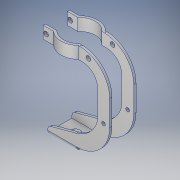
# Autodesk Inventor part: ARM
Saved by Autodesk Inventor 2018 (Build 220112000, 112)
## iProperties
Created: 2018-02-23
Part Number: ARM
Material: Aluminum 6061
Document SubType Name: Modeling
Designer: 238438
Density: 2.7 g/cm^3
Appearance: Aluminum - Flat
Mass: 2.14686 g
Surface Area: 19.7952 cm^2
Volume: 0.795133 cm^3
Author: 238438
Autodesk Inventor part; units mm, degrees
ref_plane "YZ Plane" through (0, 0, 0) normal (1, 0, 0) x (0, 1, 0)
ref_plane "XZ Plane" through (0, 0, 0) normal (0, 1, 0) x (-1, 0, 0)
ref_plane "XY Plane" through (0, 0, 0) normal (0, 0, 1) x (1, 0, 0)
sketch "Sketch1" plane through (0, 0, 0) normal (0, 1, 0) x (-1, 0, 0)
  line L0 (0, 0) -> (-12.0269, 0)
  line L1 (-12.0269, 0) -> (-12.0269, -11.1252)
  line L2 (-12.0269, -11.1252) -> (0, -11.1252)
  line L3 (0, -11.1252) -> (0, 0)
  circle A0 centre (-6.0198, -5.5626) radius 1.9876
  dimension "d0" = 12.0269
  dimension "d1" = 11.1252
  dimension "d2" = 5.5626
  dimension "d3" = 6.0198
  dimension "d4" = 3.9751
  constraints: 8 end point, 2 parallel, 1 centre point, 1 coincident, 1 horizontal, 1 perpendicular
  measures "d0" distance of L2.end L1.end
  measures "d1" distance of L1.end L0.end
  measures "d2" distance from line of L0 point (-6.02, -5.563)
  measures "d3" distance from line of L3 point (-6.02, -5.563)
  measures "d4" diameter of A0
extrude "Extrusion1" add sketch "Sketch1" along normal blind 0.9652
sketch "Sketch2" plane through (0, 0.9652, 0) normal (0, 1, 0) x (1, 0, 0)
  line L0 (0, 11.1252) -> (0, 0) projected
  line L1 (12.0269, 0) -> (12.0269, 11.1252) projected
  line L2 (0, 0) -> (12.0269, 0)
  line L3 (12.0269, 0) -> (12.0269, 0.9779)
  line L4 (12.0269, 0.9779) -> (0, 0.9779)
  line L5 (0, 0.9779) -> (0, 0)
  line L6 (12.0269, 11.1252) -> (0, 11.1252) projected
  line L7 (12.0269, 11.1252) -> (0, 11.1252)
  line L8 (0, 11.1252) -> (0, 10.1473)
  line L9 (0, 10.1473) -> (12.0269, 10.1473)
  line L10 (12.0269, 10.1473) -> (12.0269, 11.1252)
  dimension "d7" = 0.9779
  dimension "d8" = 0.9779
  constraints: 16 end point, 4 parallel, 2 horizontal, 2 perpendicular, 2 point on line
  measures "d7" distance of L3.end L2.end
  measures "d8" distance of L8.end L7.end
extrude "Extrusion2" add sketch "Sketch2" along normal blind 12.7 contours L6 L1 L9 L0 | L4 L1 L2 L0
sketch "Sketch3" plane through (0, 0, 0) normal (0, 0, 1) x (1, 0, 0)
  line L0 (0, 0.9652) -> (0, 13.6652) projected
  line L1 (0, 3.302) -> (12.0269, 6.5246)
  line L2 (12.0269, 0.9652) -> (12.0269, 13.6652) projected
  line L3 (0, 3.302) -> (12.4512, 3.302) construction
  line L4 (0, 3.302) -> (0, 13.6652)
  line L5 (0, 13.6652) -> (12.0269, 13.6652) projected
  line L6 (0, 13.6652) -> (12.0269, 13.6652)
  line L7 (12.0269, 6.5246) -> (12.0269, 13.6652)
  point P0 (0, 0)
  dimension "d11" = 15
  constraints: 10 end point, 3 collinear, 2 point on line, 1 equal length, 1 horizontal
  measures "d11" angle of L3 L1
extrude "Extrusion3" cut sketch "Sketch3" against normal through all
fillet "Fillet1" radius 1.5875 2 edges at (6.0135, 0, 0) (6.0135, 0, -11.1252)
fillet "Fillet2" radius 1.5875 2 edges at (0, 3.302, -10.6363) (0, 3.302, -0.4889)
sketch "Sketch4" plane through (12.0269, 0.9652, -0.9779) normal (1, 0, 0) x (0, 0, -1)
  arc A0 (-0.9779, 0.6223) -> (0.6096, -0.9652) centre (0.6096, 0.6223) ccw projected
  line L0 (-0.9779, 0.6223) -> (0, 0.6223)
  line L1 (0, 0) -> (0, 1.1187) projected
  arc A1 (8.5598, -0.9652) -> (10.1473, 0.6223) centre (8.5598, 0.6223) ccw projected
  line L2 (10.1473, 0.6223) -> (9.1694, 0.6223)
  line L3 (9.1694, 0) -> (9.1694, 1.1187) projected
  line L4 (9.1694, 5.5594) -> (9.1694, 2.6521) projected
  line L5 (9.1694, 0.6223) -> (9.1694, 5.5594)
  line L6 (0, 5.5594) -> (-0.9779, 5.5594) projected
  line L7 (-0.9779, 5.5594) -> (0, 5.5594)
  line L8 (0, 5.5594) -> (0, 0.6223)
  line L9 (0, 0.6223) -> (-0.9779, 0.6223)
  line L10 (-0.9779, 0.6223) -> (-0.9779, 5.5594)
  line L11 (10.1473, 2.6521) -> (10.1473, 5.5594) projected
  line L12 (9.1694, 0.6223) -> (10.1473, 0.6223)
  line L13 (10.1473, 0.6223) -> (10.1473, 5.5594)
  line L14 (10.1473, 5.5594) -> (9.1694, 5.5594)
  line L15 (9.1694, 5.5594) -> (9.1694, 0.6223)
  point P0 (-0.9779, -0.9652)
  constraints: 22 end point, 4 parallel, 3 horizontal, 3 point on line, 2 perpendicular, 1 vertical
extrude "Extrusion4" add sketch "Sketch4" along normal blind 13.97
sketch "Sketch5" plane through (12.0269, 6.5246, 0) normal (0, 1, 0) x (1, 0, 0)
  line L0 (0, 10.1473) -> (13.97, 10.1473) projected
  line L1 (13.97, 11.1252) -> (0, 11.1252)
  line L2 (0, 11.1252) -> (0, 10.1473)
  line L3 (0, 10.1473) -> (13.97, 10.1473)
  line L4 (13.97, 10.1473) -> (13.97, 11.1252)
  line L5 (0, 0.9779) -> (0, 10.1473) projected
  line L6 (0, 0) -> (13.97, 0) projected
  line L7 (0, 0.9779) -> (13.97, 0.9779)
  line L8 (13.97, 0.9779) -> (13.97, 0)
  line L9 (13.97, 0) -> (0, 0)
  line L10 (0, 0) -> (0, 0.9779)
  point P0 (-12.0269, 0)
  constraints: 16 end point, 4 parallel, 2 horizontal, 2 perpendicular
extrude "Extrusion5" add sketch "Sketch5" along normal blind 32.385
sketch "Sketch6" plane through (25.9969, 1.5875, -11.1252) normal (0, 0, -1) x (-1, 0, 0)
  line L0 (0, 0) -> (0, 37.3221) projected
  line L1 (13.97, 0) -> (25.9969, 0) projected
  arc A0 (0, 13.97) -> (13.97, 0) centre (13.97, 13.97) ccw
  line L2 (13.97, 0) -> (0, 13.97) construction
  line L3 (13.97, 0) -> (33.7266, 0) construction
  line L4 (13.97, 0) -> (0, 0) projected
  line L5 (0, 13.97) -> (0, 0)
  line L6 (0, 0) -> (13.97, 0)
  line L7 (5.08, 24.006) -> (5.08, 13.97)
  line L8 (24.8203, 2.0298) -> (13.97, 4.9371) projected
  arc A1 (5.08, 13.97) -> (13.97, 4.9371) centre (17.3693, 17.1737) ccw
  line L9 (5.08, 24.006) -> (5.08, 37.3221)
  line L10 (0, 37.3221) -> (13.97, 37.3221) projected
  line L11 (0, 37.3221) -> (5.08, 37.3221)
  line L12 (13.97, 4.9371) -> (13.97, 37.3221) projected
  line L13 (13.97, 4.9371) -> (13.97, 37.3221)
  line L14 (13.97, 37.3221) -> (5.08, 37.3221)
  point P0 (25.9969, -1.5875)
  dimension "d20" = 135
  dimension "d21" = 13.97
  dimension "d22" = 5.08
  dimension "d23" = 12.7
  constraints: 18 end point, 4 point on circle, 4 vertical, 3 perpendicular, 2 centre point, 2 point on line, 1 equal length, 1 horizontal
  measures "d20" angle of L3 L2
  measures "d21" radius of A0
  measures "d22" distance from line of L7.start L0
  measures "d23" radius of A1
extrude "Extrusion6" cut sketch "Sketch6" against normal through all
fillet "Fillet3" radius 1.5875 2 edges at (20.9169, 15.5575, -10.6363) (20.9169, 15.5575, -0.4889)
sketch "Sketch7" plane through (20.9169, 38.9096, -11.1252) normal (-1, 0, 0) x (0, 0, 1)
  line L0 (0, -23.3521) -> (0, 0) projected
  line L1 (0.9779, -23.3521) -> (0.9779, 0) projected
  line L2 (0, 0) -> (0.9779, 0)
  line L3 (0.9779, 0) -> (0.9779, -5.08)
  line L4 (0.9779, -5.08) -> (0, -5.08)
  line L5 (0, -5.08) -> (0, 0)
  line L6 (10.1473, -23.3521) -> (10.1473, 0) projected
  line L7 (11.1252, -23.3521) -> (11.1252, 0) projected
  line L8 (10.1473, 0) -> (11.1252, 0)
  line L9 (11.1252, 0) -> (11.1252, -5.08)
  line L10 (11.1252, -5.08) -> (10.1473, -5.08)
  line L11 (10.1473, -5.08) -> (10.1473, 0)
  point P0 (11.1252, -38.9096)
  dimension "d27" = 5.08
  dimension "d28" = 5.08
  constraints: 16 end point, 4 parallel, 2 horizontal, 2 perpendicular, 2 point on line
  measures "d27" distance of L2.end L3.end
  measures "d28" distance of L8.end L9.end
extrude "Extrusion7" add sketch "Sketch7" along normal blind 22.86
fillet "Fillet4" radius 6.35 2 edges at (20.9169, 33.8296, -0.4889) (20.9169, 33.8296, -10.6363)
fillet "Fillet5" radius 12.7 2 edges at (25.9969, 38.9096, -0.4889) (25.9969, 38.9096, -10.6363)
sketch "Sketch11" plane through (12.0269, 38.9096, 0) normal (0, 1, 0) x (1, 0, 0)
  line L0 (-13.97, 0) -> (-13.97, 0.9779) projected
  line L1 (-13.97, 0) -> (1.27, 0) projected
  circle A0 centre (-4.445, 5.715) radius 6.731
  line L2 (1.27, 0.9779) -> (-13.97, 0.9779) projected
  circle A1 centre (-4.445, 5.715) radius 7.7216
  line L3 (-12.0269, 0.9779) -> (0, 0.9779) projected
  line L4 (-9.2269, 0.9779) -> (-10.5428, 0.9779)
  line L5 (0, 0.9779) -> (8.8313, 0.9779) projected
  line L6 (0.3369, 0.9779) -> (1.6528, 0.9779)
  line L7 (8.8313, 10.1473) -> (0, 10.1473) projected
  line L8 (1.8778, 10.1473) -> (0.6207, 10.1473)
  line L9 (2.54, 10.1473) -> (-13.97, 10.1473) projected
  line L10 (-10.7678, 10.1473) -> (-9.5107, 10.1473)
  point P0 (-12.0269, 0)
  dimension "d56" = 9.525
  dimension "d57" = 5.715
  dimension "d58" = 13.462
  dimension "d59" = 0.9779
  dimension "d60" = 0.9906
  constraints: 8 end point, 8 point on circle, 8 point on line, 2 centre point, 2 coincident
  measures "d56" distance from line of L0 point (-4.445, 5.715)
  measures "d57" distance from line of L1 point (-4.445, 5.715)
  measures "d58" diameter of A0
  measures "d59" distance between parallel lines of L2 L1
  measures "d60" radial gap between concentric circles of A1 A0
extrude "Extrusion11" add sketch "Sketch11" against normal blind 5.08 contours A1 L2 A0 L1 | L1 A0 A1 | L1 A0 L2 L5 A1 | A1 L7 A0 L9
sketch "Sketch10" plane through (12.0269, 1.5875, -11.1252) normal (0, 0, -1) x (-1, 0, 0)
  line L0 (13.97, 37.3221) -> (13.97, 32.2421) projected
  line L1 (-1.27, 37.3221) -> (13.97, 37.3221) projected
  line L2 (-1.27, 37.3221) -> (-1.27, 37.3221) projected
  line L3 (-1.27, 32.2421) -> (-1.27, 37.3221) projected
  line L4 (-13.97, 13.97) -> (-13.97, 24.6221) projected
  arc A0 (-8.89, 14.1804) -> (-8.8313, 13.7528) centre (-7.3025, 14.1804) ccw projected
  circle A1 centre (12.7, 34.7821) radius 0.9906
  circle A2 centre (-5.08, 34.7821) radius 0.9906
  circle A3 centre (-11.43, 14.1804) radius 0.762
  point P0 (12.0269, -1.5875)
  point P1 (9.9543, 37.3221)
  dimension "d45" = 1.27
  dimension "d46" = 2.54
  dimension "d47" = 2.54
  dimension "d48" = 3.81
  dimension "d49" = 2.54
  dimension "d50" = 0
  dimension "d51" = 1.9812
  dimension "d52" = 1.9812
  dimension "d53" = 1.524
  constraints: 3 centre point, 3 coincident
  measures "d45" distance from line of L0 point (12.7, 34.782)
  measures "d46" distance from line of point (12.7, 34.782) L1
  measures "d47" distance from line of L2 point (-5.08, 34.782)
  measures "d48" distance from line of L3 point (-5.08, 34.782)
  measures "d49" distance from line of L4 point (-11.43, 14.18)
  measures "d50" vertical distance of A0.centre point (-11.43, 14.18)
  measures "d51" diameter of A1
  measures "d52" diameter of A2
  measures "d53" diameter of A3
extrude "Extrusion10" cut sketch "Sketch10" against normal through all
sketch "Sketch12" plane through (12.0269, 38.9096, 0) normal (0, 1, 0) x (1, 0, 0)
  line L0 (-13.97, 10.1473) -> (-13.97, 11.1252) projected
  line L1 (-13.97, 0) -> (1.27, 0) projected
  circle A0 centre (-4.445, 5.715) radius 6.731
  point P0 (-12.0269, 0)
  point P1 (-9.6375, 0)
  dimension "d63" = 9.525
  dimension "d64" = 5.715
  constraints: 1 centre point, 1 coincident
  measures "d63" distance from line of L0 point (-4.445, 5.715)
  measures "d64" distance from line of L1 point (-4.445, 5.715)
extrude "Extrusion12" cut sketch "Sketch12" against normal blind 5.08
body "Solid1"
